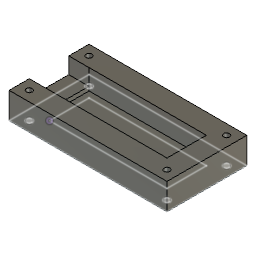
macropad (Autodesk Fusion 360 design; units mm, degrees)
part number: 2026-08-09-13-25-07-924
Autodesk Fusion 360 part; units mm, degrees
sketch "Sketch1" plane through (0, 0, 0) normal (0, 0, 1) x (1, 0, 0)
  line L0 (0, 0) -> (57.8, 0)
  line L1 (57.8, 0) -> (57.8, 19.4)
  line L2 (57.8, 19.4) -> (0, 19.4)
  line L3 (0, 19.4) -> (0, 0)
  line L4 (-10, -10) -> (67.8, -10)
  line L5 (67.8, -10) -> (67.8, 29.4)
  line L6 (67.8, 29.4) -> (-10, 29.4)
  line L7 (-10, 29.4) -> (-10, -10)
  circle A0 centre (-5, 24.4) radius 1.45
  circle A1 centre (-5, -5) radius 1.45
  circle A2 centre (62.8, -5) radius 1.45
  circle A3 centre (62.8, 24.4) radius 1.45
  dimension "d1" = 57.8
  dimension "d2" = 19.4
  dimension "d3" = 10
  dimension "d4" = 10
  dimension "d5" = 10
  dimension "d6" = 10
  dimension "d7" = 2.9
  dimension "d8" = 5
  dimension "d9" = 5
  dimension "d10" = 2.9
  dimension "d11" = 5
  dimension "d12" = 5
  dimension "d13" = 2.9
  dimension "d14" = 5
  dimension "d15" = 5
  dimension "d16" = 2.9
  dimension "d17" = 5
  dimension "d18" = 5
  constraint horizontal L0
  constraint vertical L1
  constraint horizontal L2
  constraint vertical L3
  constraint coincident L0.start L3.end
  constraint horizontal L4
  constraint vertical L5
  constraint horizontal L6
  constraint vertical L7
  measures "d1" distance of L0.start L0.end
  measures "d2" distance of L0.start L2.end
  measures "d3" distance of L3 L7
  measures "d4" distance of L0 L4
  measures "d5" distance of L1 L5
  measures "d6" distance of L2 L6
  measures "d7" diameter of A0
  measures "d8" distance of L7 A0.centre
  measures "d9" distance of L6 A0.centre
  measures "d10" diameter of A1
  measures "d11" distance of L4 A1.centre
  measures "d12" distance of L7 A1.centre
  measures "d13" diameter of A2
  measures "d14" distance of L5 A2.centre
  measures "d15" distance of L4 A2.centre
  measures "d16" diameter of A3
  measures "d17" distance of L5 A3.centre
  measures "d18" distance of L6 A3.centre
extrude "Extrude1" add sketch "Sketch1" along normal blind 13 makes body 1
extrude "Extrude2" add sketch "Sketch1" along normal blind 3 separate body contours L0 L1 L2 L3 makes body 2
sketch "Sketch2" plane through (-10, 0, 0) normal (-1, 0, 0) x (0, -1, 0)
  line L0 (-29.4, 0) -> (10, 0)
  line L1 (10, 0) -> (10, 13)
  line L2 (10, 13) -> (-29.4, 13)
  line L3 (-29.4, 13) -> (-29.4, 0)
  line L4 (-19.3698, 13) -> (0, 13)
  line L5 (0, 13) -> (0, 5)
  line L6 (0, 5) -> (-19.3698, 5)
  line L7 (-19.3698, 5) -> (-19.3698, 13)
  point P0 (-19.4, 13)
  dimension "d24" = 8
  dimension "d25" = 0.0302
  constraint horizontal L4
  constraint vertical L5
  constraint horizontal L6
  constraint vertical L7
  constraint coincident L2 L4.start
  measures "d24" distance of L4.start L6.end
  measures "d25" distance of L7 P0
extrude "Extrude3" cut sketch "Sketch2" against normal blind 21 contours L2 L4 L5 L6 L7 bodies 1
